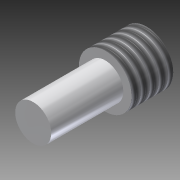
# Autodesk Inventor part: USD S1-100-B Shaft
Saved by Autodesk Inventor 2012 (Build 160160000, 160)
## iProperties
Created: 2012-07-07
Part Number: USD S1-100-B Shaft
Material: Default
Document SubType Name: Modeling
Designer: Programming Team
Density: 1 g/cm^3
Author: Programming Team
Autodesk Inventor part; units mm, degrees
ref_plane "YZ Plane" through (0, 0, 0) normal (1, 0, 0) x (0, 1, 0)
ref_plane "XZ Plane" through (0, 0, 0) normal (0, 1, 0) x (-1, 0, 0)
ref_plane "XY Plane" through (0, 0, 0) normal (0, 0, 1) x (1, 0, 0)
sketch "Sketch1" plane through (0, 0, 0) normal (0, 0, 1) x (1, 0, 0)
  circle A0 centre (0, 0) radius 4.6482
  circle A1 centre (0, 0) radius 3.175
  dimension "d0" = 9.2964
  dimension "d1" = 6.35
  constraints: 2 centre point, 2 coincident
  measures "d0" diameter of A0
  measures "d1" diameter of A1
extrude "Extrusion1" add sketch "Sketch1" against normal blind 7.3152 contours A0 | A1
extrude "Extrusion2" add sketch "Sketch1" along normal blind 12.7 contours A1
thread "Thread1" size "3/8-16 UNC" class "2A" standard "ANSI Unified Screw Threads" full length
body "Solid1"
